Autodesk Fusion 360 part; units mm, degrees
(part 7 of 7)
  arc A96 (-7.0223, -2.9045) -> (-7.5245, -2.6799) centre (-7.392, -3.0573) ccw
sketch "Sketch3 (2)" plane through (0, 0, 0) normal (0, 0, -1) x (-1, 0, 0)
component "Spur Gear (24 teeth)" placed x (1, 0, 0) y (0, 1, 0) z (0, 0, 1) at (0, 0, 0)
